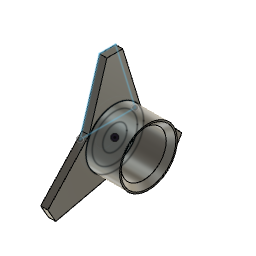
イージーペインターボトム (Autodesk Fusion 360 design; units mm, degrees)
Autodesk Fusion 360 part; units mm, degrees
note: some values were not read from the file. Set by a fixed rule: which face or edge a step refers to.
sketch "スケッチ1" plane through (0, 0, 0) normal (1, 0, 0) x (0, 1, 0)
  circle A0 centre (0, 0) radius 9.4
  circle A1 centre (0, 0) radius 12
  dimension "d1" = 18.8
  dimension "d2" = 24
  constraint coincident A0.centre A1.centre
  measures "d1" diameter of A0
  measures "d2" diameter of A1
extrude "押し出し1" add sketch "スケッチ1" along normal blind 10 makes body 1
chamfer "面取り1" distance 2 angle 45 1 edges at (10, -8.7639, 3.3992) on bodies 1
extrude "押し出し2" add sketch "スケッチ1" against normal blind 3 contours A0 | A1 bodies 1
sketch "スケッチ2" plane through (0, 0, 0) normal (1, 0, 0) x (0, 1, 0)
  circle A0 centre (0, 0) radius 5
  dimension "d8" = 10
  constraint coincident A0.centre origin
  measures "d8" diameter of A0
extrude "押し出し3" cut sketch "スケッチ2" against normal blind 35 bodies 1
sketch "スケッチ3" plane through (-3, 0, 0) normal (-1, 0, 0) x (0, -1, 0)
  circle A0 centre (0, 0) radius 5
  circle A1 centre (0, 0) radius 12
  line L0 (-3.311, 30.2948) -> (3.311, 30.2948)
  line L1 (3.311, 30.2948) -> (11.4786, 3.4988)
  line L2 (-3.311, 30.2948) -> (-11.4786, 3.4988)
  line L3 (-11.4786, 3.4988) -> (11.4786, 3.4988)
  constraint horizontal L0
  constraint coincident A1 L1.end
  constraint tangent A1 L1
  constraint coincident A1 L2.end
  constraint tangent A1 L2
  constraint horizontal L3
extrude "押し出し4" add sketch "スケッチ3" against normal blind 3 separate body contours A0 A1 L3 | A1 L0 L1 L2 picked at (6.6282, 7.0035) makes body 2
move_face "面を移動1" to x (0.99863, 0, 0.052336) y (0, 1, 0) z (-0.052336, 0, 0.99863) at (0, 0, 0) 1 faces at (0, -5.7382, 12.722) on bodies 2
pattern_circular "C パターン1" count 3 over 360 about axis through (1.75, 0, 0) along (1, 0, 0) of bodies 2 makes body 3 at (-0.6709, -8.2982, -11.2291) makes body 4 at (-0.6709, 13.8738, -1.5718)
move_face "面を移動2" to x (1, 0, 0) y (0, 1, 0) z (0, 0, 1) at (4, 0, 0) 2 faces at (9.3333, -10.68, 1.0687) (10, 10.8498, 4.5633) on bodies 1
combine "結合1" operation add target body 1 tool bodies 2 3 4
delete_face "面を削除1" 1 faces at (-0.2983, -0.4042, -12.0855) on bodies 1
delete_face "面を削除2" 1 faces at (-0.3118, 1.8062, -11.8995) on bodies 1
delete_face "面を削除3" 1 faces at (-0.3118, 11.2083, 4.3855) on bodies 1
delete_face "面を削除4" 1 faces at (-0.3118, 9.4021, 7.5139) on bodies 1
delete_face "面を削除5" 1 faces at (-0.3118, -11.2083, 4.3855) on bodies 1
delete_face "面を削除6" 1 faces at (-0.3118, -9.4021, 7.5139) on bodies 1
move_face "面を移動3" by (0.9986, -0.0453, -0.0262) 3 faces at (-1.2681, -20.9819, -12.0505) (-1.268, -0.1318, 24.1943) (-1.2677, 20.8201, -12.3152) on bodies 1
delete_face "面を削除7" 1 faces at (-0.2707, 21.0083, -12.0025) on bodies 1
delete_face "面を削除8" 1 faces at (-0.2703, -0.2758, 24.187) on bodies 1
delete_face "面を削除9" 1 faces at (1.6354, 0, 24.1965) on bodies 1
extrude "押し出し5" add sketch "スケッチ3" against normal blind 3 separate body contours A1 L0 L1 L2 makes body 5
pattern_circular "C パターン2" count 3 over 360 about axis through (1.75, 0, 0) along (1, 0, 0) of bodies 5 makes body 6 at (-3, -20.7952, -12.3522) makes body 7 at (-3, 20.7952, -12.3522)
combine "結合2" operation add target body 1 tool bodies 6 5
combine "結合3" operation add target body 1 tool bodies 7
